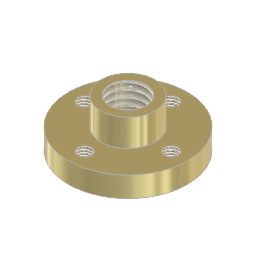
_Lead Screw Connector.f1a2c122-9b56-4b04-ac3e-5ceb7d299708 (Autodesk Fusion 360 design; units mm, degrees)
Autodesk Fusion 360 part; units mm, degrees
sketch "Sketch1" plane through (0, 0, 0) normal (0, 0, 1) x (1, 0, 0)
  circle A0 centre (0, 0) radius 11
  circle A1 centre (0, 0) radius 4
  dimension "d1_4" = 22
  dimension "d2_4" = 8
  constraint coincident A0.centre A1.centre
  constraint concentric A0 A1
  measures "d1_4" diameter of A0
  measures "d2_4" diameter of A1
extrude "Extrude1" add sketch "Sketch1" along normal blind 3.8
sketch "Sketch2" plane through (0, 0, 3.8) normal (0, 0, 1) x (-1, 0, 0)
  circle A0 centre (0, 0) radius 4
  circle A1 centre (0, 0) radius 11
  circle A2 centre (0, 0) radius 5
  dimension "d5_1" = 10
  constraint coincident A0.centre A1.centre
  measures "d5_1" diameter of A2
extrude "Extrude2" add sketch "Sketch2" along normal blind 5 contours A2
sketch "Sketch3" plane through (0, 0, 0) normal (0, 0, -1) x (1, 0, 0)
  circle A0 centre (0, 0) radius 4
  circle A1 centre (0, 0) radius 11
  circle A2 centre (0, 0) radius 5
  dimension "d8_1" = 10
  constraint coincident A0.centre A1.centre
  measures "d8_1" diameter of A2
extrude "Extrude3" add sketch "Sketch3" along normal blind 1.7 contours A2
sketch "Sketch4" plane through (0, 0, 3.8) normal (0, 0, 1) x (-1, 0, 0)
  circle A0 centre (0, 0) radius 5
  circle A1 centre (0, 0) radius 11
  circle A2 centre (0, 0) radius 8 construction
  circle A3 centre (0, 8) radius 1.4
  line L0 (0, 0) -> (-15, 0) construction
  circle A4 centre (-8, 0) radius 1.4
  circle A5 centre (8, 0) radius 1.4
  circle A6 centre (0, -8) radius 1.4
  dimension "d11_1" = 16
  dimension "d12_1" = 2.8
  dimension "d13_1" = 2.8
  dimension "d14_1" = 2.8
  dimension "d15_1" = 2.8
  constraint coincident A0.centre A1.centre
  constraint coincident A2 A3.centre
  constraint horizontal L0
  constraint coincident A2 A4.centre
  constraint coincident L0 A4.centre
  constraint coincident A2 A5.centre
  constraint coincident A2 A6.centre
  measures "d11_1" diameter of A2
  measures "d12_1" diameter of A3
  measures "d13_1" diameter of A4
  measures "d14_1" diameter of A5
  measures "d15_1" diameter of A6
hole "Hole1" at (8, 0, 3.8) at (0, 8, 3.8) at (0, -8, 3.8) at (-8, 0, 3.8) direction (0, 0, -1) diameter 2.529 depth 3 tip angle 118
thread "Thread1" "ISO Metric profile 3.0 M3x0.5 M3x0.5 6H" major diameter 3.086 minor diameter 2.529 pitch 0.5 angle 60 resizes the face on face at (8.063, -1.2629, 2.8) on face at (0.063, 6.7371, 2.8) on face at (0.063, -9.2629, 2.8) on face at (-7.937, -1.2629, 2.8)
thread "Thread2" "ISO Metric profile 8.0 M8x1.25 M8x1.25 6H" major diameter 8.17 minor diameter 6.7795 pitch 1.25 angle 60 resizes the face on face at (3.9801, -0.3983, 3.6333)
equation "d9_1 = 10.5 mm - 8.8 mm"
